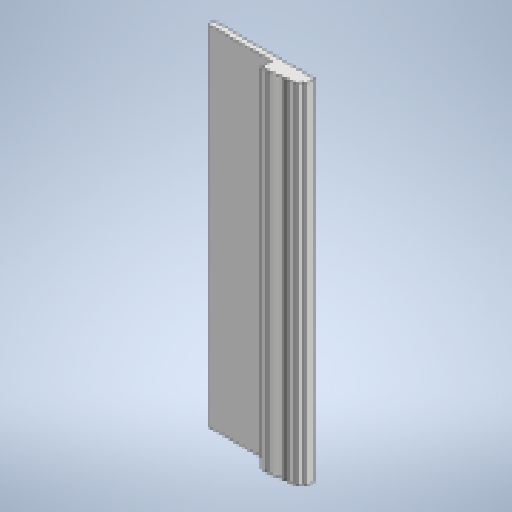
# Autodesk Inventor part: moulding
Saved by Autodesk Inventor 2023 (Build 270158000, 158)
## iProperties
Created: 2022-12-04
Part Number: moulding
Material: Generic
Document SubType Name: Modeling
Designer: shrey
Density: 1 g/cm^3
Appearance: Default
Author: shrey
Autodesk Inventor part; units mm, degrees
ref_plane "YZ Plane" through (0, 0, 0) normal (1, 0, 0) x (0, 1, 0)
ref_plane "XZ Plane" through (0, 0, 0) normal (0, 1, 0) x (-1, 0, 0)
ref_plane "XY Plane" through (0, 0, 0) normal (0, 0, 1) x (1, 0, 0)
sketch "Sketch1" plane through (0, 0, 0) normal (0, 1, 0) x (-1, 0, 0)
  line L0 (0, 0) -> (-144.4624, 0) construction
  line L1 (20.965, -35.9101) -> (-87.0678, -35.9101) construction
  line L2 (-87.0678, -35.9101) -> (-87.0678, 30.1756) construction
  line L3 (-87.0678, 30.1756) -> (20.965, 30.1756) construction
  line L4 (20.965, 30.1756) -> (20.965, -35.9101) construction
  line L5 (-98.2096, -3.929) -> (-103.1995, -4.2465) construction
  line L6 (-98.2096, -3.929) -> (-101.5606, 48.7236) construction
  line L7 (-103.1995, -4.2465) -> (-107.6572, 65.7945) construction
  line L8 (0, 0) -> (-9.9035, 0)
  line L9 (-9.9035, -0.8852) -> (-9.9035, 0)
  spline S0 degree 4 poles (-9.9035, -0.8852) (-13.0419, -1.1842) (-21.2538, 1.0327) (-27.8606, -5.346) (-33.2586, -4.0317) (-34.8616, -3.7545) knots 0 0 0 0 0 0.558486 0.866888 0.866888 0.866888 0.866888 0.866888
  line L10 (-34.8616, -3.7545) -> (-37.2153, -3.929)
  line L11 (-32.3863, -4.1825) -> (-37.3369, -3.3265) construction
  arc A0 (-32.9001, -4.1709) -> (-36.8491, -3.488) centre (-39.3648, -29.7961) ccw construction
  line L12 (-37.2153, -3.929) -> (-37.2153, -4.9671)
  line L13 (-37.2153, -4.9671) -> (-41.1207, -5.3635)
  spline S1 degree 2 poles (-41.1207, -5.3635) (-45.6353, -4.1273) (-50.1475, -5.6677) knots 0 0 0 1 1 1
  spline S2 degree 2 poles (-50.1475, -5.6677) (-53.2023, -5.0279) (-57.1879, -6.1401) knots 0 0 0 1 1 1
  line L14 (0, 0) -> (0, -18.5)
  line L15 (0, -18.5) -> (-57.1879, -18.5)
  line L16 (-57.1879, -18.5) -> (-57.1879, -6.1401)
  line L17 (-57.1879, -18.5) -> (111, -18.5)
  line L18 (111, -18.5) -> (111, -28.5)
  line L19 (111, -28.5) -> (-57.1879, -28.5)
  line L20 (-57.1879, -28.5) -> (-57.1879, -18.5)
  line L21 (-57.1879, -28.5) -> (-64.1879, -28.5)
  line L22 (-64.1879, -28.5) -> (-64.1879, -13.1401)
  line L23 (-64.1879, -13.1401) -> (-57.1879, -13.1401)
  line L24 (-57.1879, -13.1401) -> (-57.1879, -28.5)
  point P0 (-57.1205, -12.0308)
  point P1 (-24.1668, -2.2709)
  point P2 (-30.6059, -4.0877)
  point P3 (-45.613, -4.8207)
  point P4 (-53.1813, -5.4511)
  dimension "d100" = 66.0857
  dimension "d113" = 5
  dimension "d119" = 30.1756
  dimension "d121" = 20.965
  dimension "d140" = 18.5
  dimension "d144" = 111
  dimension "d145" = 10
  dimension "d146" = 7
  dimension "d147" = 7
  constraints: 42 end point, 7 perpendicular, 4 parallel, 4 vertical, 3 horizontal, 2 midpoint, 2 point on line, 1 centre point, 1 point on circle, 29 other
  measures "d100" distance of L3.end L1.start
  measures "d113" distance between parallel lines of L7 L6
  measures "d119" vertical distance of L3.end L0.start
  measures "d121" horizontal distance of L3.end L0.start
  measures "d140" distance of L0.start L14.end
  measures "d144" distance between parallel lines of L18 L14
  measures "d145" distance between parallel lines of L17 L19
  measures "d146" distance of L22.end L23.end
  measures "d147" distance from line of L16.end L23
extrude "Extrusion1" add sketch "Sketch1" along normal mid plane 609.6
equation "\"d100\" = 186.046 * scale"
equation "\"d113\" = 14.0761 * scale"
equation "\"scale\" = 0.355211"
body "Solid1"
